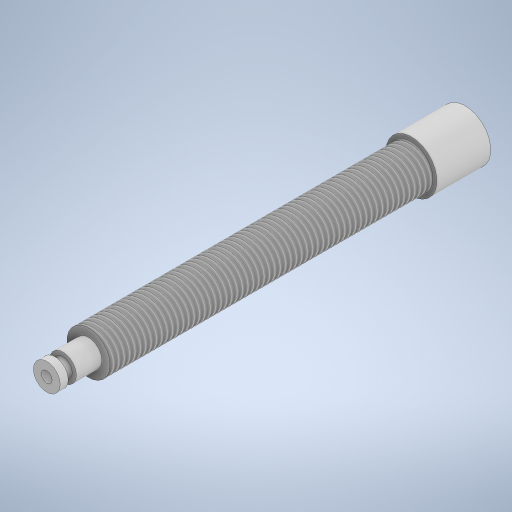
# Autodesk Inventor part: Trapezspindle
Saved by Autodesk Inventor 2024 (Build 280153000, 153)
## iProperties
Created: 2023-05-10
Part Number: Trapezspindle
Material: Generic
Document SubType Name: Modeling
Designer: dell
Density: 1 g/cm^3
Appearance: Default
Author: dell
Autodesk Inventor part; units mm, degrees
ref_plane "YZ Plane" through (0, 0, 0) normal (1, 0, 0) x (0, 1, 0)
ref_plane "XZ Plane" through (0, 0, 0) normal (0, 1, 0) x (-1, 0, 0)
sketch "Sketch1" plane through (0, 0, 0) normal (0, 0, 1) x (1, 0, 0)
  circle A0 centre (0, 0) radius 8
  dimension "d0" = 16
  constraints: 1 centre point, 1 coincident
  measures "d0" diameter of A0
extrude "Extrusion1" add sketch "Sketch1" along normal blind 120
sketch "Sketch2" plane through (0, 0, 120) normal (0, 0, 1) x (1, 0, 0)
  circle A0 centre (0, 0) radius 5
  dimension "d3" = 10
  constraints: 1 centre point, 1 coincident
  measures "d3" diameter of A0
extrude "Extrusion2" add sketch "Sketch2" along normal blind 9.5
sketch "Sketch3" plane through (0, 0, 0) normal (0, 0, -1) x (-1, 0, 0)
  circle A0 centre (0, 0) radius 9.5
  dimension "d44" = 19
  constraints: 1 centre point, 1 coincident
  measures "d44" diameter of A0
extrude "Extrusion3" add sketch "Sketch3" along normal blind 20
sketch "Sketch5" plane through (0, 0, 129.5) normal (0, 0, 1) x (1, 0, 0)
  circle A0 centre (0, 0) radius 5
  constraints: 1 centre point, 1 coincident
extrude "Extrusion4" add sketch "Sketch5" along normal blind 6
sketch "Sketch8" plane through (0, 0, 135.5) normal (0, 0, 1) x (1, 0, 0)
  circle A0 centre (0, 0) radius 5 projected
  circle A1 centre (0, 0) radius 2
  dimension "d27" = 4
  constraints: 1 centre point, 1 coincident
  measures "d27" diameter of A1
extrude "Extrusion7" cut sketch "Sketch8" against normal blind 160 contours A1
sketch "Sketch10" plane through (0, 0, 135.5) normal (0, 0, 1) x (1, 0, 0)
  circle A0 centre (0, 0) radius 5 projected
  point P0 (5, 0)
  constraints: 1 horizontal alignment, 1 other
sketch "Sketch11" plane through (0, 0, 135.5) normal (0, 0, 1) x (1, 0, 0)
  point P0 (0, 0)
ref_plane "Work Plane1" through (5, 0, 135.5) normal (0, 1, 0) x (-1, 0, 0)
sketch "Sketch12" plane through (5, 0, 135.5) normal (0, 1, 0) x (-1, 0, 0)
  arc A0 (1.5, -6) -> (1.5, -3) centre (1.5, -4.5) ccw
  line L0 (13, -15.5) -> (-3, -15.5) projected
  line L1 (3, 0) -> (3, -155.5) projected
  line L2 (5, -186.6) -> (5, 31.1) projected
  line L3 (0, -15.5) -> (0, 0) projected
  arc A1 (1.5, -6) -> (1.5, -3) centre (1.5, -4.5) ccw
  line L4 (1.5, -3) -> (0, -3)
  line L5 (0, -15.5) -> (0, 0) projected
  line L6 (0, -6) -> (1.5, -6)
  line L7 (0, -15.5) -> (0, 0) projected
  point P0 (5, -135.5)
  point P1 (3, -4.5)
  point P2 (3, -4.5)
  point P3 (0, -6)
  dimension "d46" = 11
  dimension "d54" = 3.5
  dimension "d55" = 3
  constraints: 6 point on circle, 4 end point, 4 point on line, 3 tangent, 2 centre point, 2 perpendicular, 1 coincident
  measures "d46" distance from line of L0 A0.centre
  measures "d54" distance from line of L2 A0.centre
  measures "d55" diameter of A1
revolve "Revolution1" cut sketch "Sketch12" angle 360 about axis through (0, 0, 120) along (0, 0, 1) contours L6 L3 L4 A0
thread "Thread1" size "M16x2" class "6g" standard "ANSI Metric M Profile" full length
body "Solid1"
